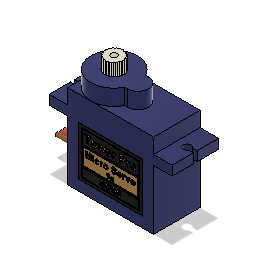
SG90 (Autodesk Fusion 360 design; units mm, degrees)
Autodesk Fusion 360 part; units mm, degrees
note: some values were not read from the file. Chosen so that the rebuilt part matches the saved one: which bodies a step acts on.
(part 1 of 2)
sketch "Sketch1" plane through (0, 0, 0) normal (0, 1, 0) x (1, 0, 0)
  line L0 (0, 0) -> (22.7, 0)
  line L1 (22.7, 0) -> (22.7, 12.3)
  line L2 (22.7, 12.3) -> (0, 12.3)
  line L3 (0, 12.3) -> (0, 0)
  dimension "d1" = 22.7
  dimension "d2" = 12.3
  constraint coincident L0.start L3.end
  constraint horizontal L0
  constraint perpendicular L0 L1
  constraint perpendicular L1 L2
  constraint perpendicular L0 L3
  measures "d1" distance of L0.start L0.end
  measures "d2" distance of L0.end L1.end
extrude "Extrude1" add sketch "Sketch1" along normal blind 22.3 makes body 1
sketch "Sketch2" plane through (0, 0, 0) normal (0, -1, 0) x (1, 0, 0)
  line L0 (0, 0) -> (0, -12.3)
  line L1 (0, -12.3) -> (22.7, -12.3)
  line L2 (22.7, -12.3) -> (22.7, 0)
  line L3 (22.7, 0) -> (0, 0)
  circle A0 centre (1.4, -1.7) radius 0.9
  circle A1 centre (1.4, -10.6) radius 0.9
  circle A2 centre (21.3, -1.7) radius 0.9
  circle A3 centre (21.3, -10.6) radius 0.9
  dimension "d9" = 1.8
  dimension "d10" = 1.8
  dimension "d11" = 1.8
  dimension "d12" = 1.8
  measures "d9" diameter of A0
  measures "d10" diameter of A1
  measures "d11" diameter of A2
  measures "d12" diameter of A3
extrude "Extrude2" cut sketch "Sketch2" against normal blind 1 contours A0 | A1 | A2 | A3 bodies 1
sketch "Sketch3" plane through (0, 1, 0) normal (0, -1, 0) x (1, 0, 0)
  circle A0 centre (1.4, -1.7) radius 0.9
  circle A1 centre (1.4, -1.7) radius 0.875
  dimension "d15" = 1.75
  constraint concentric A0 A1
  measures "d15" diameter of A1
extrude "Extrude3" add sketch "Sketch3" along normal blind 1 separate body contours A1 makes body 2
sketch "Sketch4" plane through (0, 0, 0) normal (0, -1, 0) x (1, 0, 0)
  circle A0 centre (1.4, -1.7) radius 0.875
  line L0 (1.9, -1.7) -> (1.9, -1.55)
  line L1 (0.9, -1.55) -> (0.9, -1.85)
  line L2 (1.9, -1.85) -> (1.9, -1.7)
  line L3 (1.4, -2.2) -> (1.55, -2.2)
  line L4 (1.55, -1.2) -> (1.25, -1.2)
  line L5 (1.25, -2.2) -> (1.4, -2.2)
  line L6 (0.9, -1.85) -> (1.25, -1.85)
  line L7 (1.55, -1.85) -> (1.9, -1.85)
  line L8 (1.25, -1.2) -> (1.25, -1.55)
  line L9 (1.25, -1.85) -> (1.25, -2.2)
  line L10 (1.9, -1.55) -> (1.55, -1.55)
  line L11 (1.25, -1.55) -> (0.9, -1.55)
  line L12 (1.55, -2.2) -> (1.55, -1.85)
  line L13 (1.55, -1.55) -> (1.55, -1.2)
  dimension "d18" = 0.15
  dimension "d19" = 0.3
  dimension "d20" = 0.15
  dimension "d21" = 0.3
  constraint perpendicular L0 L10
  constraint perpendicular L1 L10
  constraint perpendicular L1 L6
  constraint perpendicular L6 L12
  constraint perpendicular L4 L12
  constraint perpendicular L6 L8
  constraint coincident L6.end L8
  constraint collinear L6 L7
  constraint coincident L8.end L10
  constraint collinear L8 L9
  constraint coincident L10.end L12
  constraint collinear L10 L11
  constraint collinear L12 L13
  measures "d18" distance of L0.start L0.end
  measures "d19" distance of L1.start L1.end
  measures "d20" distance of L3.start L3.end
  measures "d21" distance of L4.start L4.end
extrude "Extrude4" cut sketch "Sketch4" against normal blind 0.5 contours L0 L1 L2 L3 L4 L5 L6 L7 L8 L9 L10 L11 L12 L13 bodies 2
fillet "Fillet1" radius 0.3 1 edges at (0.5842, 0, -2.0164) on bodies 2
pattern_linear "R-Pattern1" count 2 spacing 19.9 along (1, 0, 0) count 2 spacing 8.9 along (0, 0, -1) of bodies 2 makes body 3 at (20.721, 0.5333, -2.3561) makes body 4 at (2.2739, 0.5333, -10.6436) makes body 5 at (20.721, 0.5333, -11.2561)
sketch "Sketch5" plane through (0, 22.3, 0) normal (0, 1, 0) x (-1, 0, 0)
  line L0 (0, -12.3) -> (0, 0)
  line L1 (0, 0) -> (-22.7, 0)
  line L2 (-22.7, 0) -> (-22.7, -12.3)
  line L3 (-22.7, -12.3) -> (0, -12.3)
  line L4 (-12.45, -8.9) -> (-11.6509, -8.9)
  line L5 (-12.45, -3.4) -> (-11.6509, -3.4)
  arc A0 (-11.6509, -8.9) -> (-11.6509, -3.4) centre (-6.15, -6.15) ccw
  arc A1 (-12.45, -3.4) -> (-12.45, -8.9) centre (-12.45, -6.15) ccw
  line L6 (-12.3, -6.15) -> (-12.45, -6.15)
  dimension "d31" = 6.3
  dimension "d32" = 5.5
  constraint tangent L3 A0
  constraint coincident A1.centre L6.end
  constraint tangent L4 A1
  constraint tangent L5 A1
  measures "d31" distance of A0.centre A1.centre
  measures "d32" diameter of A1
extrude "Extrude5" add sketch "Sketch5" along normal blind 4.2 contours L4 L5 A0 A1 bodies 1
sketch "Sketch6" plane through (0, 26.5, 0) normal (0, 1, 0) x (-1, 0, 0)
  arc A0 (-12.45, -3.4) -> (-12.45, -8.9) centre (-12.45, -6.15) ccw
  line L0 (-12.45, -8.9) -> (-11.6509, -8.9)
  arc A1 (-11.6509, -8.9) -> (-11.6509, -3.4) centre (-6.15, -6.15) ccw
  line L1 (-11.6509, -3.4) -> (-12.45, -3.4)
  circle A2 centre (-6.15, -6.15) radius 2.5
  dimension "d35" = 5
  constraint concentric A1 A2
  measures "d35" diameter of A2
extrude "Extrude6" cut sketch "Sketch6" against normal blind 2 contours A2 bodies 1
sketch "Sketch7" plane through (0, 24.5, 0) normal (0, 1, 0) x (-1, 0, 0)
  circle A0 centre (-6.15, -6.15) radius 2.5
  line L0 (-6.15, -6.15) -> (-3.7, -6.15) construction
  line L1 (-5.8174, -8.3753) -> (-6.15, -8.6)
  line L2 (-6.15, -8.6) -> (-6.4826, -8.3753)
  line L3 (-5.1763, -8.1784) -> (-5.4278, -8.4912)
  line L4 (-5.4278, -8.4912) -> (-5.8119, -8.3744)
  line L5 (-4.6217, -7.8013) -> (-4.7699, -8.1743)
  line L6 (-4.7699, -8.1743) -> (-5.1712, -8.176)
  line L7 (-4.2028, -7.2774) -> (-4.2345, -7.6776)
  line L8 (-4.2345, -7.6776) -> (-4.6176, -7.7975)
  line L9 (-3.957, -6.6534) -> (-3.8694, -7.0451)
  line L10 (-3.8694, -7.0451) -> (-4.2, -7.2726)
  line L11 (-3.9061, -5.9847) -> (-3.7069, -6.3331)
  line L12 (-3.7069, -6.3331) -> (-3.9558, -6.6479)
  line L13 (-4.0545, -5.3306) -> (-3.7614, -5.6048)
  line L14 (-3.7614, -5.6048) -> (-3.9065, -5.9791)
  line L15 (-4.3891, -4.7493) -> (-4.0282, -4.925)
  line L16 (-4.0282, -4.925) -> (-4.0566, -5.3254)
  line L17 (-4.8802, -4.2925) -> (-4.4836, -4.354)
  line L18 (-4.4836, -4.354) -> (-4.3926, -4.745)
  line L19 (-5.4841, -4.0008) -> (-5.087, -3.9426)
  line L20 (-5.087, -3.9426) -> (-4.8848, -4.2894)
  line L21 (-6.1472, -3.9) -> (-5.7848, -3.7274)
  line L22 (-5.7848, -3.7274) -> (-5.4895, -3.9991)
  line L23 (-6.8105, -3.9991) -> (-6.5152, -3.7274)
  line L24 (-6.5152, -3.7274) -> (-6.1528, -3.9)
  line L25 (-7.4152, -4.2894) -> (-7.213, -3.9426)
  line L26 (-7.213, -3.9426) -> (-6.8159, -4.0008)
  line L27 (-7.9074, -4.745) -> (-7.8164, -4.354)
  line L28 (-7.8164, -4.354) -> (-7.4198, -4.2925)
  line L29 (-8.2434, -5.3254) -> (-8.2718, -4.925)
  line L30 (-8.2718, -4.925) -> (-7.9109, -4.7493)
  line L31 (-8.3935, -5.9791) -> (-8.5386, -5.6048)
  line L32 (-8.5386, -5.6048) -> (-8.2455, -5.3306)
  line L33 (-8.3442, -6.6479) -> (-8.5931, -6.3331)
  line L34 (-8.5931, -6.3331) -> (-8.3939, -5.9847)
  line L35 (-8.1, -7.2726) -> (-8.4306, -7.0451)
  line L36 (-8.4306, -7.0451) -> (-8.343, -6.6534)
  line L37 (-7.6824, -7.7975) -> (-8.0655, -7.6776)
  line L38 (-8.0655, -7.6776) -> (-8.0972, -7.2774)
  line L39 (-7.1288, -8.176) -> (-7.5301, -8.1743)
  line L40 (-7.5301, -8.1743) -> (-7.6783, -7.8013)
  line L41 (-6.4881, -8.3744) -> (-6.8722, -8.4912)
  line L42 (-6.8722, -8.4912) -> (-7.1237, -8.1784)
  arc A1 (-6.4881, -8.3744) -> (-6.4826, -8.3753) centre (-6.15, -6.15) ccw
  arc A2 (-7.1288, -8.176) -> (-7.1237, -8.1784) centre (-6.15, -6.15) ccw
  arc A3 (-7.6824, -7.7975) -> (-7.6783, -7.8013) centre (-6.15, -6.15) ccw
  arc A4 (-5.8174, -8.3753) -> (-5.8119, -8.3744) centre (-6.15, -6.15) ccw
  arc A5 (-5.1763, -8.1784) -> (-5.1712, -8.176) centre (-6.15, -6.15) ccw
  arc A6 (-4.6217, -7.8013) -> (-4.6176, -7.7975) centre (-6.15, -6.15) ccw
  arc A7 (-4.2028, -7.2774) -> (-4.2, -7.2726) centre (-6.15, -6.15) ccw
  arc A8 (-3.957, -6.6534) -> (-3.9558, -6.6479) centre (-6.15, -6.15) ccw
  arc A9 (-3.9061, -5.9847) -> (-3.9065, -5.9791) centre (-6.15, -6.15) ccw
  arc A10 (-4.0545, -5.3306) -> (-4.0566, -5.3254) centre (-6.15, -6.15) ccw
  arc A11 (-4.3891, -4.7493) -> (-4.3926, -4.745) centre (-6.15, -6.15) ccw
  arc A12 (-4.8802, -4.2925) -> (-4.8848, -4.2894) centre (-6.15, -6.15) ccw
  arc A13 (-5.4841, -4.0008) -> (-5.4895, -3.9991) centre (-6.15, -6.15) ccw
  arc A14 (-6.1472, -3.9) -> (-6.1528, -3.9) centre (-6.15, -6.15) ccw
  arc A15 (-6.8105, -3.9991) -> (-6.8159, -4.0008) centre (-6.15, -6.15) ccw
  arc A16 (-7.4152, -4.2894) -> (-7.4198, -4.2925) centre (-6.15, -6.15) ccw
  arc A17 (-7.9074, -4.745) -> (-7.9109, -4.7493) centre (-6.15, -6.15) ccw
  arc A18 (-8.2434, -5.3254) -> (-8.2455, -5.3306) centre (-6.15, -6.15) ccw
  arc A19 (-8.3935, -5.9791) -> (-8.3939, -5.9847) centre (-6.15, -6.15) ccw
  arc A20 (-8.3442, -6.6479) -> (-8.343, -6.6534) centre (-6.15, -6.15) ccw
  arc A21 (-8.1, -7.2726) -> (-8.0972, -7.2774) centre (-6.15, -6.15) ccw
  dimension "d39" = 4.5
  dimension "d43" = 360
  constraint concentric A0 A4
  constraint horizontal L0
  constraint concentric A1 A4
  constraint concentric A2 A4
  constraint concentric A3 A4
  constraint concentric A4 A5
  constraint concentric A5 A6
  constraint concentric A6 A7
  constraint concentric A7 A8
  constraint concentric A8 A9
  constraint concentric A9 A10
  constraint concentric A10 A11
  constraint concentric A11 A12
  constraint concentric A12 A13
  constraint concentric A13 A14
  constraint concentric A14 A15
  constraint concentric A15 A16
  constraint concentric A16 A17
  constraint concentric A17 A18
  constraint concentric A18 A19
  constraint concentric A19 A20
  constraint concentric A20 A21
  measures "d39" diameter of A4
extrude "Extrude7" add sketch "Sketch7" along normal blind 5.2 separate body contours L1 L2 L3 L4 L5 L6 L7 L8 L9 L10 L11 L12 L13 L14 L15 L16 L17 L18 L19 L20 L21 L22 L23 L24 L25 L26 L27 L28 L29 L30 L31 L32 L33 L34 L35 L36 L37 L38 L39 L40 L41 L42 A1 A2 A3 A4 A5 A6 A7 A8 A9 A10 A11 A12 A13 A14 A15 A16 A17 A18 A19 A20 A21 makes body 6
sketch "Sketch8" plane through (0, 29.7, 0) normal (0, 1, 0) x (-1, 0, 0)
  line L0 (-8.4306, -7.0451) -> (-8.1, -7.2726)
  arc A0 (-8.1, -7.2726) -> (-8.0972, -7.2774) centre (-6.15, -6.15) ccw
  line L1 (-8.0972, -7.2774) -> (-8.0655, -7.6776)
  line L2 (-8.0655, -7.6776) -> (-7.6824, -7.7975)
  arc A1 (-7.6824, -7.7975) -> (-7.6783, -7.8013) centre (-6.15, -6.15) ccw
  line L3 (-7.6783, -7.8013) -> (-7.5301, -8.1743)
  line L4 (-7.5301, -8.1743) -> (-7.1288, -8.176)
  arc A2 (-7.1288, -8.176) -> (-7.1237, -8.1784) centre (-6.15, -6.15) ccw
  line L5 (-7.1237, -8.1784) -> (-6.8722, -8.4912)
  line L6 (-6.8722, -8.4912) -> (-6.4881, -8.3744)
  arc A3 (-6.4881, -8.3744) -> (-6.4826, -8.3753) centre (-6.15, -6.15) ccw
  line L7 (-6.4826, -8.3753) -> (-6.15, -8.6)
  line L8 (-6.15, -8.6) -> (-5.8174, -8.3753)
  arc A4 (-5.8174, -8.3753) -> (-5.8119, -8.3744) centre (-6.15, -6.15) ccw
  line L9 (-5.8119, -8.3744) -> (-5.4278, -8.4912)
  line L10 (-5.4278, -8.4912) -> (-5.1763, -8.1784)
  arc A5 (-5.1763, -8.1784) -> (-5.1712, -8.176) centre (-6.15, -6.15) ccw
  line L11 (-5.1712, -8.176) -> (-4.7699, -8.1743)
  line L12 (-4.7699, -8.1743) -> (-4.6217, -7.8013)
  arc A6 (-4.6217, -7.8013) -> (-4.6176, -7.7975) centre (-6.15, -6.15) ccw
  line L13 (-4.6176, -7.7975) -> (-4.2345, -7.6776)
  line L14 (-4.2345, -7.6776) -> (-4.2028, -7.2774)
  arc A7 (-4.2028, -7.2774) -> (-4.2, -7.2726) centre (-6.15, -6.15) ccw
  line L15 (-4.2, -7.2726) -> (-3.8694, -7.0451)
  line L16 (-3.8694, -7.0451) -> (-3.957, -6.6534)
  arc A8 (-3.957, -6.6534) -> (-3.9558, -6.6479) centre (-6.15, -6.15) ccw
  line L17 (-3.9558, -6.6479) -> (-3.7069, -6.3331)
  line L18 (-3.7069, -6.3331) -> (-3.9061, -5.9847)
  arc A9 (-3.9061, -5.9847) -> (-3.9065, -5.9791) centre (-6.15, -6.15) ccw
  line L19 (-3.9065, -5.9791) -> (-3.7614, -5.6048)
  line L20 (-3.7614, -5.6048) -> (-4.0545, -5.3306)
  arc A10 (-4.0545, -5.3306) -> (-4.0566, -5.3254) centre (-6.15, -6.15) ccw
  line L21 (-4.0566, -5.3254) -> (-4.0282, -4.925)
  line L22 (-4.0282, -4.925) -> (-4.3891, -4.7493)
  arc A11 (-4.3891, -4.7493) -> (-4.3926, -4.745) centre (-6.15, -6.15) ccw
  line L23 (-4.3926, -4.745) -> (-4.4836, -4.354)
  line L24 (-4.4836, -4.354) -> (-4.8802, -4.2925)
  arc A12 (-4.8802, -4.2925) -> (-4.8848, -4.2894) centre (-6.15, -6.15) ccw
  line L25 (-4.8848, -4.2894) -> (-5.087, -3.9426)
  line L26 (-5.087, -3.9426) -> (-5.4841, -4.0008)
  arc A13 (-5.4841, -4.0008) -> (-5.4895, -3.9991) centre (-6.15, -6.15) ccw
  line L27 (-5.4895, -3.9991) -> (-5.7848, -3.7274)
  line L28 (-5.7848, -3.7274) -> (-6.1472, -3.9)
  arc A14 (-6.1472, -3.9) -> (-6.1528, -3.9) centre (-6.15, -6.15) ccw
  line L29 (-6.1528, -3.9) -> (-6.5152, -3.7274)
  line L30 (-6.5152, -3.7274) -> (-6.8105, -3.9991)
  arc A15 (-6.8105, -3.9991) -> (-6.8159, -4.0008) centre (-6.15, -6.15) ccw
  line L31 (-6.8159, -4.0008) -> (-7.213, -3.9426)
  line L32 (-7.213, -3.9426) -> (-7.4152, -4.2894)
  arc A16 (-7.4152, -4.2894) -> (-7.4198, -4.2925) centre (-6.15, -6.15) ccw
  line L33 (-7.4198, -4.2925) -> (-7.8164, -4.354)
  line L34 (-7.8164, -4.354) -> (-7.9074, -4.745)
  arc A17 (-7.9074, -4.745) -> (-7.9109, -4.7493) centre (-6.15, -6.15) ccw
  line L35 (-7.9109, -4.7493) -> (-8.2718, -4.925)
  line L36 (-8.2718, -4.925) -> (-8.2434, -5.3254)
  arc A18 (-8.2434, -5.3254) -> (-8.2455, -5.3306) centre (-6.15, -6.15) ccw
  line L37 (-8.2455, -5.3306) -> (-8.5386, -5.6048)
  line L38 (-8.5386, -5.6048) -> (-8.3935, -5.9791)
  arc A19 (-8.3935, -5.9791) -> (-8.3939, -5.9847) centre (-6.15, -6.15) ccw
  line L39 (-8.3939, -5.9847) -> (-8.5931, -6.3331)
  line L40 (-8.5931, -6.3331) -> (-8.3442, -6.6479)
  arc A20 (-8.3442, -6.6479) -> (-8.343, -6.6534) centre (-6.15, -6.15) ccw
  line L41 (-8.343, -6.6534) -> (-8.4306, -7.0451)
  circle A21 centre (-6.15, -6.15) radius 0.8
  dimension "d46" = 1.6
  constraint concentric A0 A21
  measures "d46" diameter of A21
extrude "Extrude8" cut sketch "Sketch8" against normal blind 4 contours A21 bodies 6
sketch "Sketch9" plane through (22.7, 0, 0) normal (1, 0, 0) x (0, 0, -1)
  line L0 (0, 0) -> (12.3, 0)
  line L1 (12.3, 0) -> (12.3, 22.3)
  line L2 (12.3, 22.3) -> (0, 22.3)
  line L3 (0, 22.3) -> (0, 0)
  line L4 (12.3, 22.3) -> (12.3, 15.8)
  line L5 (12.3, 15.8) -> (0, 15.8)
  line L6 (0, 15.8) -> (0, 18.3)
  line L7 (0, 18.3) -> (12.3, 18.3256)
  line L8 (12.3, 18.3256) -> (12.3, 15.8)
  dimension "d49" = 6.5
  dimension "d50" = 2.5
  constraint coincident L1.end L2.start
  constraint perpendicular L2 L4
  constraint coincident L3 L5.end
  constraint perpendicular L3 L5
  constraint perpendicular L5 L6
  constraint coincident L1 L7.end
  measures "d49" distance of L1.end L4.end
  measures "d50" distance of L5.end L6.end
extrude "Extrude9" add sketch "Sketch9" along normal blind 4.9 contours L1 L3 L4 L5 L6 L7 L8 bodies 1
sketch "Sketch10" plane through (0, 18.2999, 0.038) normal (0, 0.999998, 0.002078) x (1, 0, 0)
  line L0 (22.7, 12.3381) -> (22.7, 0.038)
  line L1 (22.7, 0.038) -> (27.6, 0.038)
  line L2 (27.6, 0.038) -> (27.6, 12.3381)
  line L3 (27.6, 12.3381) -> (22.7, 12.3381)
  line L4 (27.6, 6.188) -> (27.6, 6.688)
  line L5 (27.6, 6.688) -> (26.316, 6.688)
  line L6 (27.6, 6.188) -> (27.6, 5.688)
  line L7 (27.6, 5.688) -> (26.316, 5.688)
  arc A0 (26.316, 6.688) -> (26.316, 5.688) centre (25.45, 6.188) ccw
  dimension "d53" = 2.15
  dimension "d54" = 2
  dimension "d55" = 0.5
  dimension "d56" = 0.5
  constraint midpoint L2 L4.start
  constraint perpendicular L4 L5
  constraint perpendicular L2 L7
  measures "d53" distance of L4.start A0.centre
  measures "d54" diameter of A0
  measures "d55" distance of L4.start L4.end
  measures "d56" distance of L4.start L6.end
extrude "Extrude10" cut sketch "Sketch10" against normal blind 7 contours L2 L4 L5 L6 L7 A0 bodies 1
sketch "Sketch11" plane through (0, 15.8, 0) normal (0, -1, 0) x (1, 0, 0)
  line L0 (26.316, -5.6552) -> (27.6, -5.6552)
  line L1 (27.6, -5.6552) -> (27.6, 0)
  line L2 (27.6, 0) -> (22.7, 0)
  line L3 (22.7, 0) -> (22.7, -12.3)
  line L4 (22.7, -12.3) -> (27.6, -12.3)
  line L5 (27.6, -12.3) -> (27.6, -6.6552)
  line L6 (27.6, -6.6552) -> (26.316, -6.6552)
  ellipse E0 centre (25.45, -6.1552) end of major axis (25.45, -7.1552) minor radius 1 (26.316, -5.6552) -> (26.316, -6.6552) ccw
  line L7 (23.7, -1) -> (22.7, -1)
  line L8 (23.7, -11.3) -> (22.7, -11.3)
  spline S0 degree 3 poles (23.7, -7.1235) (23.7918, -7.2893) (23.908, -7.443) (24.0431, -7.5767) (24.5836, -8.1117) (25.4438, -8.2949) (26.1554, -8.0267) (26.3127, -7.9674) (26.4625, -7.8882) (26.6, -7.7915) knots 5.21775 5.21775 5.21775 5.21775 5.502936 5.502936 5.502936 6.643656 6.643656 6.643656 6.895789 6.895789 6.895789 6.895789
  line L9 (26.6, -11.3) -> (26.6, -7.7915)
  spline S1 degree 3 poles (26.6, -4.5189) (26.2218, -4.2531) (25.748, -4.1241) (25.2866, -4.1619) (24.633, -4.2155) (24.0163, -4.6152) (23.7, -5.187) knots 2.528989 2.528989 2.528989 2.528989 3.223367 3.223367 3.223367 4.207028 4.207028 4.207028 4.207028
  line L10 (26.6, -1) -> (23.7, -1)
  line L11 (26.6, -4.5189) -> (26.6, -1)
  arc A0 (26.6, -4.5189) -> (26.6, -7.7915) centre (25.45, -6.1552) ccw
  line L12 (23.7, -11.3) -> (26.6, -11.3)
  line L13 (22.7, -11.3) -> (22.7, -1)
  constraint coincident L3 L7.end
  constraint perpendicular L3 L7
  constraint coincident L3 L8.end
  constraint perpendicular L3 L8
  constraint perpendicular L9 L12
extrude "Extrude11" cut sketch "Sketch11" against normal blind 1 contours L3 L7 L8 S0 L9 S1 L10 L11 A0 L12 L13 bodies 1
ref_plane "WorkPlane1" through (11.35, 0, 0) normal (1, 0, 0) x (0, 1, 0)
mirror "Mirror1" about plane through (11.35, 0, 0) normal (1, 0, 0) of "Extrude9"
mirror "Mirror2" about plane through (11.35, 0, 0) normal (1, 0, 0) of "Extrude10"
mirror "Mirror3" about plane through (11.35, 0, 0) normal (1, 0, 0) of "Extrude11"
sketch "Sketch12" plane through (0, 0, 0) normal (0, 0, 1) x (1, 0, 0)
  line L0 (0, 0) -> (22.7, 0)
  line L1 (22.7, 0) -> (22.7, 15.8)
  line L2 (22.7, 15.8) -> (27.6, 15.8)
  line L3 (27.6, 15.8) -> (27.6, 18.3)
  line L4 (27.6, 18.3) -> (22.7, 18.3)
  line L5 (22.7, 18.3) -> (22.7, 22.3)
  line L6 (22.7, 22.3) -> (6.15, 22.3)
  line L7 (6.15, 22.3) -> (0, 22.3)
  line L8 (0, 22.3) -> (0, 18.3)
  line L9 (0, 18.3) -> (-4.9, 18.3)
  line L10 (-4.9, 18.3) -> (-4.9, 15.8)
  line L11 (-4.9, 15.8) -> (0, 15.8)
  line L12 (0, 15.8) -> (0, 0)
  line L13 (11.35, 0) -> (19.85, 0)
  line L14 (19.85, 15.8) -> (2.85, 15.8)
  line L15 (19.85, 15.8) -> (19.85, 2.8)
  line L16 (19.85, 2.8) -> (2.85, 2.8)
  line L17 (2.85, 2.8) -> (2.85, 15.8)
  dimension "d69" = 8.5
  dimension "d70" = 13
  dimension "d71" = 17
  constraint midpoint L0 L13.start
  constraint parallel L0 L13
  constraint perpendicular L14 L15
  constraint perpendicular L15 L16
  constraint perpendicular L14 L17
  measures "d69" distance of L13.start L13.end
  measures "d70" distance of L14.start L15.end
  measures "d71" distance of L15.end L16.end
extrude "Extrude12" add sketch "Sketch12" along normal blind 0.05 separate body contours L14 L15 L16 L17 makes body 7
sketch "Sketch13" plane through (0, 0, 0.05) normal (0, 0, 1) x (1, 0, 0)
  line L0 (19.85, 15.8) -> (2.85, 15.8)
  line L1 (2.85, 15.8) -> (2.85, 2.8)
  line L2 (2.85, 2.8) -> (19.85, 2.8)
  line L3 (19.85, 2.8) -> (19.85, 15.8)
  line L4 (19.05, 9.3) -> (19.05, 15.05)
  line L5 (19.05, 15.05) -> (3.65, 15.05)
  line L6 (3.65, 15.05) -> (3.65, 3.55)
  line L7 (3.65, 3.55) -> (19.05, 3.55)
  line L8 (19.05, 3.55) -> (19.05, 9.3)
  line L9 (3.65, 15.05) -> (3.85, 15.05)
  line L10 (3.85, 3.75) -> (18.85, 3.75)
  line L11 (18.85, 14.85) -> (3.85, 14.85)
  line L12 (3.85, 14.85) -> (3.85, 11.35)
  line L13 (3.85, 11.35) -> (18.85, 11.35)
  line L14 (18.85, 11.15) -> (3.85, 11.15)
  line L15 (3.85, 14.85) -> (3.85, 11.35)
  line L16 (18.85, 11.35) -> (18.85, 14.85)
  line L17 (18.85, 3.75) -> (18.85, 6.05)
  line L18 (18.85, 6.05) -> (3.85, 6.05)
  line L19 (3.85, 6.25) -> (18.85, 6.25)
  line L20 (18.85, 3.75) -> (18.85, 6.05)
  line L21 (18.85, 6.25) -> (18.85, 11.15)
  line L22 (3.85, 11.15) -> (3.85, 6.25)
  line L23 (3.85, 6.05) -> (3.85, 3.75)
  line L24 (3.85, 11.15) -> (4.15, 11.15)
  line L25 (4.15, 10.85) -> (4.15, 6.55)
  line L26 (4.15, 10.85) -> (18.55, 10.85)
  line L27 (18.55, 10.85) -> (18.55, 6.55)
  line L28 (18.55, 6.55) -> (4.15, 6.55)
  dimension "d75" = 5.75
  dimension "d76" = 15.4
  dimension "d77" = 11.5
  dimension "d78" = 15.4
  dimension "d79" = 0.2
  dimension "d83" = 3.5
  dimension "d84" = 0.2
  dimension "d85" = 2.3
  dimension "d86" = 0.2
  dimension "d87" = 0.3
  dimension "d88" = 0.3
  constraint perpendicular L4 L5
  constraint perpendicular L5 L6
  constraint perpendicular L6 L7
  constraint horizontal L9
  constraint perpendicular L7 L15
  constraint perpendicular L8 L10
  constraint perpendicular L5 L20
  constraint perpendicular L11 L15
  constraint perpendicular L11 L12
  constraint coincident L13.end L20
  constraint perpendicular L13 L20
  constraint coincident L14.end L15
  constraint perpendicular L14 L15
  constraint collinear L15 L22
  constraint collinear L16 L20
  constraint perpendicular L10 L17
  constraint coincident L18.end L22
  constraint perpendicular L18 L22
  constraint coincident L19.end L20
  constraint perpendicular L19 L20
  constraint collinear L20 L21
  constraint collinear L22 L23
  constraint perpendicular L22 L24
  constraint perpendicular L19 L25
  constraint perpendicular L21 L26
  constraint perpendicular L19 L27
  constraint perpendicular L25 L28
  measures "d75" distance of L4.start L4.end
  measures "d76" distance of L4.end L5.end
  measures "d77" distance of L5.end L6.end
  measures "d78" distance of L6.end L7.end
  measures "d79" distance of L5.end L9.end
  measures "d83" distance of L11.end L12.end
  measures "d84" distance of L13.end L14.start
  measures "d85" distance of L10.end L17.end
  measures "d86" distance of L18.end L19.start
  measures "d87" distance of L14.end L24.end
  measures "d88" distance of L24.end L25.start
extrude "Extrude13" add sketch "Sketch13" along normal blind 0.05 contours L4 L5 L6 L7 L8 L9 | L25 L26 L27 L28 bodies 7
sketch "Sketch14" plane through (0, 0, 0.05) normal (0, 0, 1) x (1, 0, 0)
  line L0 (18.85, 14.85) -> (3.85, 14.85)
  line L1 (3.85, 14.85) -> (3.85, 11.35)
  line L2 (3.85, 11.35) -> (18.85, 11.35)
  line L3 (18.85, 11.35) -> (18.85, 14.85)
  line L4 (5.1924, 12.1) -> (5.1924, 13.7617)
  line L5 (5.1924, 13.7617) -> (4.599, 13.7617)
  line L6 (4.599, 13.7617) -> (4.599, 14.1)
  line L7 (4.599, 14.1) -> (6.1883, 14.1)
  line L8 (6.1883, 14.1) -> (6.1883, 13.7617)
  line L9 (6.1883, 13.7617) -> (5.5962, 13.7617)
  line L10 (5.5962, 13.7617) -> (5.5962, 12.1)
  line L11 (5.5962, 12.1) -> (5.1924, 12.1)
  spline S0 degree 2 poles (6.3575, 12.8449) (6.3575, 13.0359) (6.4516, 13.2146) knots 0 0 0 1 1 1
  spline S1 degree 2 poles (6.4516, 13.2146) (6.5458, 13.3933) (6.7177, 13.4874) knots 0 0 0 1 1 1
  spline S2 degree 2 poles (6.7177, 13.4874) (6.8909, 13.5816) (7.1038, 13.5816) knots 0 0 0 1 1 1
  spline S3 degree 2 poles (7.1038, 13.5816) (7.4325, 13.5816) (7.6426, 13.3674) knots 0 0 0 1 1 1
  spline S4 degree 2 poles (7.6426, 13.3674) (7.8527, 13.1546) (7.8527, 12.8285) knots 0 0 0 1 1 1
  spline S5 degree 2 poles (7.8527, 12.8285) (7.8527, 12.4997) (7.6399, 12.2828) knots 0 0 0 1 1 1
  spline S6 degree 2 poles (7.6399, 12.2828) (7.4284, 12.0673) (7.1065, 12.0673) knots 0 0 0 1 1 1
  spline S7 degree 2 poles (7.1065, 12.0673) (6.9073, 12.0673) (6.7259, 12.1573) knots 0 0 0 1 1 1
  spline S8 degree 2 poles (6.7259, 12.1573) (6.5458, 12.2473) (6.4516, 12.4206) knots 0 0 0 1 1 1
  spline S9 degree 2 poles (6.4516, 12.4206) (6.3575, 12.5952) (6.3575, 12.8449) knots 0 0 0 1 1 1
  spline S10 degree 2 poles (6.7504, 12.8244) (6.7504, 12.6089) (6.8527, 12.4943) knots 0 0 0 1 1 1
  spline S11 degree 2 poles (6.8527, 12.4943) (6.955, 12.3797) (7.1051, 12.3797) knots 0 0 0 1 1 1
  spline S12 degree 2 poles (7.1051, 12.3797) (7.2552, 12.3797) (7.3561, 12.4943) knots 0 0 0 1 1 1
  spline S13 degree 2 poles (7.3561, 12.4943) (7.4585, 12.6089) (7.4585, 12.8271) knots 0 0 0 1 1 1
  spline S14 degree 2 poles (7.4585, 12.8271) (7.4585, 13.04) (7.3561, 13.1546) knots 0 0 0 1 1 1
  spline S15 degree 2 poles (7.3561, 13.1546) (7.2552, 13.2692) (7.1051, 13.2692) knots 0 0 0 1 1 1
  spline S16 degree 2 poles (7.1051, 13.2692) (6.955, 13.2692) (6.8527, 13.1546) knots 0 0 0 1 1 1
  spline S17 degree 2 poles (6.8527, 13.1546) (6.7504, 13.04) (6.7504, 12.8244) knots 0 0 0 1 1 1
  line L12 (8.423, 12.1) -> (7.9646, 13.5488)
  line L13 (7.9646, 13.5488) -> (8.337, 13.5488)
  line L14 (8.337, 13.5488) -> (8.6085, 12.5993)
  line L15 (8.6085, 12.5993) -> (8.8582, 13.5488)
  line L16 (8.8582, 13.5488) -> (9.2279, 13.5488)
  line L17 (9.2279, 13.5488) -> (9.4694, 12.5993)
  line L18 (9.4694, 12.5993) -> (9.7463, 13.5488)
  line L19 (9.7463, 13.5488) -> (10.1242, 13.5488)
  line L20 (10.1242, 13.5488) -> (9.659, 12.1)
  line L21 (9.659, 12.1) -> (9.2907, 12.1)
  line L22 (9.2907, 12.1) -> (9.041, 13.0318)
  line L23 (9.041, 13.0318) -> (8.7954, 12.1)
  line L24 (8.7954, 12.1) -> (8.423, 12.1)
  line L25 (11.1651, 12.5611) -> (11.5471, 12.497)
  spline S18 degree 2 poles (11.5471, 12.497) (11.4735, 12.2869) (11.3138, 12.1764) knots 0 0 0 1 1 1
  spline S19 degree 2 poles (11.3138, 12.1764) (11.1556, 12.0673) (10.9168, 12.0673) knots 0 0 0 1 1 1
  spline S20 degree 2 poles (10.9168, 12.0673) (10.5389, 12.0673) (10.3575, 12.3142) knots 0 0 0 1 1 1
  spline S21 degree 2 poles (10.3575, 12.3142) (10.2143, 12.512) (10.2143, 12.8135) knots 0 0 0 1 1 1
  spline S22 degree 2 poles (10.2143, 12.8135) (10.2143, 13.1737) (10.4025, 13.3769) knots 0 0 0 1 1 1
  spline S23 degree 2 poles (10.4025, 13.3769) (10.5908, 13.5816) (10.8786, 13.5816) knots 0 0 0 1 1 1
  spline S24 degree 2 poles (10.8786, 13.5816) (11.202, 13.5816) (11.3889, 13.3674) knots 0 0 0 1 1 1
  spline S25 degree 2 poles (11.3889, 13.3674) (11.5758, 13.1546) (11.5676, 12.7139) knots 0 0 0 1 1 1
  line L26 (11.5676, 12.7139) -> (10.6072, 12.7139)
  spline S26 degree 2 poles (10.6072, 12.7139) (10.6113, 12.5434) (10.6999, 12.4479) knots 0 0 0 1 1 1
  spline S27 degree 2 poles (10.6999, 12.4479) (10.7886, 12.3538) (10.9209, 12.3538) knots 0 0 0 1 1 1
  spline S28 degree 2 poles (10.9209, 12.3538) (11.011, 12.3538) (11.0724, 12.4029) knots 0 0 0 1 1 1
  spline S29 degree 2 poles (11.0724, 12.4029) (11.1338, 12.452) (11.1651, 12.5611) knots 0 0 0 1 1 1
  spline S30 degree 2 poles (11.187, 12.9486) (11.1829, 13.115) (11.101, 13.201) knots 0 0 0 1 1 1
  spline S31 degree 2 poles (11.101, 13.201) (11.0192, 13.2883) (10.9018, 13.2883) knots 0 0 0 1 1 1
  spline S32 degree 2 poles (10.9018, 13.2883) (10.7763, 13.2883) (10.6945, 13.1969) knots 0 0 0 1 1 1
  spline S33 degree 2 poles (10.6945, 13.1969) (10.6126, 13.1055) (10.614, 12.9486) knots 0 0 0 1 1 1
  line L27 (10.614, 12.9486) -> (11.187, 12.9486)
  line L28 (12.247, 12.1) -> (11.8636, 12.1)
  line L29 (11.8636, 12.1) -> (11.8636, 13.5488)
  line L30 (11.8636, 13.5488) -> (12.2197, 13.5488)
  line L31 (12.2197, 13.5488) -> (12.2197, 13.3428)
  spline S34 degree 2 poles (12.2197, 13.3428) (12.3111, 13.4888) (12.3834, 13.5352) knots 0 0 0 1 1 1
  spline S35 degree 2 poles (12.3834, 13.5352) (12.4571, 13.5816) (12.5499, 13.5816) knots 0 0 0 1 1 1
  spline S36 degree 2 poles (12.5499, 13.5816) (12.6808, 13.5816) (12.8023, 13.5093) knots 0 0 0 1 1 1
  line L32 (12.8023, 13.5093) -> (12.6836, 13.175)
  spline S37 degree 2 poles (12.6836, 13.175) (12.5867, 13.2378) (12.5035, 13.2378) knots 0 0 0 1 1 1
  spline S38 degree 2 poles (12.5035, 13.2378) (12.423, 13.2378) (12.3671, 13.1928) knots 0 0 0 1 1 1
  spline S39 degree 2 poles (12.3671, 13.1928) (12.3111, 13.1491) (12.2784, 13.0332) knots 0 0 0 1 1 1
  spline S40 degree 2 poles (12.2784, 13.0332) (12.247, 12.9172) (12.247, 12.5475) knots 0 0 0 1 1 1
  line L33 (12.247, 12.5475) -> (12.247, 12.1)
  line L34 (13.7463, 12.1) -> (13.7463, 14.1)
  line L35 (13.7463, 14.1) -> (14.3943, 14.1)
  spline S41 degree 2 poles (14.3943, 14.1) (14.7627, 14.1) (14.8746, 14.07) knots 0 0 0 1 1 1
  spline S42 degree 2 poles (14.8746, 14.07) (15.0465, 14.025) (15.1624, 13.8735) knots 0 0 0 1 1 1
  spline S43 degree 2 poles (15.1624, 13.8735) (15.2784, 13.7235) (15.2784, 13.4847) knots 0 0 0 1 1 1
  spline S44 degree 2 poles (15.2784, 13.4847) (15.2784, 13.3005) (15.2115, 13.175) knots 0 0 0 1 1 1
  spline S45 degree 2 poles (15.2115, 13.175) (15.1447, 13.0495) (15.041, 12.9772) knots 0 0 0 1 1 1
  spline S46 degree 2 poles (15.041, 12.9772) (14.9387, 12.9063) (14.8323, 12.8831) knots 0 0 0 1 1 1
  spline S47 degree 2 poles (14.8323, 12.8831) (14.6877, 12.8544) (14.4134, 12.8544) knots 0 0 0 1 1 1
  line L36 (14.4134, 12.8544) -> (14.1501, 12.8544)
  line L37 (14.1501, 12.8544) -> (14.1501, 12.1)
  line L38 (14.1501, 12.1) -> (13.7463, 12.1)
  line L39 (14.1501, 13.7617) -> (14.1501, 13.1941)
  line L40 (14.1501, 13.1941) -> (14.3711, 13.1941)
  spline S48 degree 2 poles (14.3711, 13.1941) (14.6099, 13.1941) (14.6904, 13.2255) knots 0 0 0 1 1 1
  spline S49 degree 2 poles (14.6904, 13.2255) (14.7709, 13.2569) (14.8159, 13.3237) knots 0 0 0 1 1 1
  spline S50 degree 2 poles (14.8159, 13.3237) (14.8623, 13.3906) (14.8623, 13.4793) knots 0 0 0 1 1 1
  spline S51 degree 2 poles (14.8623, 13.4793) (14.8623, 13.5884) (14.7982, 13.6593) knots 0 0 0 1 1 1
  spline S52 degree 2 poles (14.7982, 13.6593) (14.734, 13.7303) (14.6358, 13.748) knots 0 0 0 1 1 1
  spline S53 degree 2 poles (14.6358, 13.748) (14.5635, 13.7617) (14.3452, 13.7617) knots 0 0 0 1 1 1
  line L41 (14.3452, 13.7617) -> (14.1501, 13.7617)
  line L42 (15.9741, 12.1) -> (15.5908, 12.1)
  line L43 (15.5908, 12.1) -> (15.5908, 13.5488)
  line L44 (15.5908, 13.5488) -> (15.9469, 13.5488)
  line L45 (15.9469, 13.5488) -> (15.9469, 13.3428)
  spline S54 degree 2 poles (15.9469, 13.3428) (16.0383, 13.4888) (16.1106, 13.5352) knots 0 0 0 1 1 1
  spline S55 degree 2 poles (16.1106, 13.5352) (16.1842, 13.5816) (16.277, 13.5816) knots 0 0 0 1 1 1
  spline S56 degree 2 poles (16.277, 13.5816) (16.408, 13.5816) (16.5294, 13.5093) knots 0 0 0 1 1 1
  line L46 (16.5294, 13.5093) -> (16.4107, 13.175)
  spline S57 degree 2 poles (16.4107, 13.175) (16.3138, 13.2378) (16.2306, 13.2378) knots 0 0 0 1 1 1
  spline S58 degree 2 poles (16.2306, 13.2378) (16.1501, 13.2378) (16.0942, 13.1928) knots 0 0 0 1 1 1
  spline S59 degree 2 poles (16.0942, 13.1928) (16.0383, 13.1491) (16.0055, 13.0332) knots 0 0 0 1 1 1
  spline S60 degree 2 poles (16.0055, 13.0332) (15.9741, 12.9172) (15.9741, 12.5475) knots 0 0 0 1 1 1
  line L47 (15.9741, 12.5475) -> (15.9741, 12.1)
  spline S61 degree 2 poles (16.6058, 12.8449) (16.6058, 13.0359) (16.6999, 13.2146) knots 0 0 0 1 1 1
  spline S62 degree 2 poles (16.6999, 13.2146) (16.7941, 13.3933) (16.966, 13.4874) knots 0 0 0 1 1 1
  spline S63 degree 2 poles (16.966, 13.4874) (17.1392, 13.5816) (17.352, 13.5816) knots 0 0 0 1 1 1
  spline S64 degree 2 poles (17.352, 13.5816) (17.6808, 13.5816) (17.8909, 13.3674) knots 0 0 0 1 1 1
  spline S65 degree 2 poles (17.8909, 13.3674) (18.101, 13.1546) (18.101, 12.8285) knots 0 0 0 1 1 1
  spline S66 degree 2 poles (18.101, 12.8285) (18.101, 12.4997) (17.8882, 12.2828) knots 0 0 0 1 1 1
  spline S67 degree 2 poles (17.8882, 12.2828) (17.6767, 12.0673) (17.3548, 12.0673) knots 0 0 0 1 1 1
  spline S68 degree 2 poles (17.3548, 12.0673) (17.1556, 12.0673) (16.9741, 12.1573) knots 0 0 0 1 1 1
  spline S69 degree 2 poles (16.9741, 12.1573) (16.7941, 12.2473) (16.6999, 12.4206) knots 0 0 0 1 1 1
  spline S70 degree 2 poles (16.6999, 12.4206) (16.6058, 12.5952) (16.6058, 12.8449) knots 0 0 0 1 1 1
  spline S71 degree 2 poles (16.9987, 12.8244) (16.9987, 12.6089) (17.101, 12.4943) knots 0 0 0 1 1 1
  spline S72 degree 2 poles (17.101, 12.4943) (17.2033, 12.3797) (17.3534, 12.3797) knots 0 0 0 1 1 1
  spline S73 degree 2 poles (17.3534, 12.3797) (17.5035, 12.3797) (17.6044, 12.4943) knots 0 0 0 1 1 1
  spline S74 degree 2 poles (17.6044, 12.4943) (17.7068, 12.6089) (17.7068, 12.8271) knots 0 0 0 1 1 1
  spline S75 degree 2 poles (17.7068, 12.8271) (17.7068, 13.04) (17.6044, 13.1546) knots 0 0 0 1 1 1
  spline S76 degree 2 poles (17.6044, 13.1546) (17.5035, 13.2692) (17.3534, 13.2692) knots 0 0 0 1 1 1
  spline S77 degree 2 poles (17.3534, 13.2692) (17.2033, 13.2692) (17.101, 13.1546) knots 0 0 0 1 1 1
  spline S78 degree 2 poles (17.101, 13.1546) (16.9987, 13.04) (16.9987, 12.8244) knots 0 0 0 1 1 1
  line L48 (8.5877, 4.6206) -> (8.902, 4.6512)
  spline S79 degree 2 poles (8.902, 4.6512) (8.9304, 4.4929) (9.0166, 4.4187) knots 0 0 0 1 1 1
  spline S80 degree 2 poles (9.0166, 4.4187) (9.1039, 4.3445) (9.2512, 4.3445) knots 0 0 0 1 1 1
  spline S81 degree 2 poles (9.2512, 4.3445) (9.4073, 4.3445) (9.4859, 4.41) knots 0 0 0 1 1 1
  spline S82 degree 2 poles (9.4859, 4.41) (9.5656, 4.4765) (9.5656, 4.5649) knots 0 0 0 1 1 1
  spline S83 degree 2 poles (9.5656, 4.5649) (9.5656, 4.6217) (9.5317, 4.661) knots 0 0 0 1 1 1
  spline S84 degree 2 poles (9.5317, 4.661) (9.499, 4.7014) (9.416, 4.7308) knots 0 0 0 1 1 1
  spline S85 degree 2 poles (9.416, 4.7308) (9.3593, 4.7505) (9.1574, 4.8007) knots 0 0 0 1 1 1
  spline S86 degree 2 poles (9.1574, 4.8007) (8.8976, 4.8651) (8.7928, 4.9589) knots 0 0 0 1 1 1
  spline S87 degree 2 poles (8.7928, 4.9589) (8.6455, 5.091) (8.6455, 5.2809) knots 0 0 0 1 1 1
  spline S88 degree 2 poles (8.6455, 5.2809) (8.6455, 5.4031) (8.7143, 5.509) knots 0 0 0 1 1 1
  spline S89 degree 2 poles (8.7143, 5.509) (8.7841, 5.616) (8.914, 5.6716) knots 0 0 0 1 1 1
  spline S90 degree 2 poles (8.914, 5.6716) (9.045, 5.7273) (9.2294, 5.7273) knots 0 0 0 1 1 1
  spline S91 degree 2 poles (9.2294, 5.7273) (9.5306, 5.7273) (9.6823, 5.5952) knots 0 0 0 1 1 1
  spline S92 degree 2 poles (9.6823, 5.5952) (9.8351, 5.4632) (9.8428, 5.2427) knots 0 0 0 1 1 1
  line L49 (9.8428, 5.2427) -> (9.5197, 5.2285)
  spline S93 degree 2 poles (9.5197, 5.2285) (9.499, 5.3518) (9.4302, 5.4053) knots 0 0 0 1 1 1
  spline S94 degree 2 poles (9.4302, 5.4053) (9.3626, 5.4599) (9.2261, 5.4599) knots 0 0 0 1 1 1
  spline S95 degree 2 poles (9.2261, 5.4599) (9.0853, 5.4599) (9.0057, 5.402) knots 0 0 0 1 1 1
  spline S96 degree 2 poles (9.0057, 5.402) (8.9544, 5.3649) (8.9544, 5.3027) knots 0 0 0 1 1 1
  spline S97 degree 2 poles (8.9544, 5.3027) (8.9544, 5.246) (9.0024, 5.2056) knots 0 0 0 1 1 1
  spline S98 degree 2 poles (9.0024, 5.2056) (9.0635, 5.1543) (9.2993, 5.0986) knots 0 0 0 1 1 1
  spline S99 degree 2 poles (9.2993, 5.0986) (9.535, 5.043) (9.6474, 4.9829) knots 0 0 0 1 1 1
  spline S100 degree 2 poles (9.6474, 4.9829) (9.7609, 4.924) (9.8242, 4.8203) knots 0 0 0 1 1 1
  spline S101 degree 2 poles (9.8242, 4.8203) (9.8886, 4.7177) (9.8886, 4.566) knots 0 0 0 1 1 1
  spline S102 degree 2 poles (9.8886, 4.566) (9.8886, 4.4285) (9.8122, 4.3085) knots 0 0 0 1 1 1
  spline S103 degree 2 poles (9.8122, 4.3085) (9.7358, 4.1884) (9.5961, 4.1295) knots 0 0 0 1 1 1
  spline S104 degree 2 poles (9.5961, 4.1295) (9.4564, 4.0716) (9.248, 4.0716) knots 0 0 0 1 1 1
  spline S105 degree 2 poles (9.248, 4.0716) (8.9445, 4.0716) (8.7819, 4.2113) knots 0 0 0 1 1 1
  spline S106 degree 2 poles (8.7819, 4.2113) (8.6193, 4.3521) (8.5877, 4.6206) knots 0 0 0 1 1 1
  line L50 (10.9047, 4.6883) -> (10.9047, 4.9578)
  line L51 (10.9047, 4.9578) -> (11.601, 4.9578)
  line L52 (11.601, 4.9578) -> (11.601, 4.3205)
  spline S107 degree 2 poles (11.601, 4.3205) (11.4995, 4.2222) (11.3063, 4.1469) knots 0 0 0 1 1 1
  spline S108 degree 2 poles (11.3063, 4.1469) (11.1143, 4.0727) (10.9167, 4.0727) knots 0 0 0 1 1 1
  spline S109 degree 2 poles (10.9167, 4.0727) (10.6657, 4.0727) (10.4791, 4.1775) knots 0 0 0 1 1 1
  spline S110 degree 2 poles (10.4791, 4.1775) (10.2924, 4.2834) (10.1986, 4.4787) knots 0 0 0 1 1 1
  spline S111 degree 2 poles (10.1986, 4.4787) (10.1047, 4.6752) (10.1047, 4.9055) knots 0 0 0 1 1 1
  spline S112 degree 2 poles (10.1047, 4.9055) (10.1047, 5.1554) (10.2095, 5.3497) knots 0 0 0 1 1 1
  spline S113 degree 2 poles (10.2095, 5.3497) (10.3143, 5.5439) (10.5162, 5.6476) knots 0 0 0 1 1 1
  spline S114 degree 2 poles (10.5162, 5.6476) (10.6701, 5.7273) (10.8993, 5.7273) knots 0 0 0 1 1 1
  spline S115 degree 2 poles (10.8993, 5.7273) (11.1972, 5.7273) (11.3642, 5.6018) knots 0 0 0 1 1 1
  spline S116 degree 2 poles (11.3642, 5.6018) (11.5323, 5.4774) (11.5803, 5.2569) knots 0 0 0 1 1 1
  line L53 (11.5803, 5.2569) -> (11.2594, 5.1969)
  spline S117 degree 2 poles (11.2594, 5.1969) (11.2256, 5.3147) (11.1317, 5.3824) knots 0 0 0 1 1 1
  spline S118 degree 2 poles (11.1317, 5.3824) (11.0389, 5.4512) (10.8993, 5.4512) knots 0 0 0 1 1 1
  spline S119 degree 2 poles (10.8993, 5.4512) (10.6875, 5.4512) (10.562, 5.3169) knots 0 0 0 1 1 1
  spline S120 degree 2 poles (10.562, 5.3169) (10.4376, 5.1827) (10.4376, 4.9186) knots 0 0 0 1 1 1
  spline S121 degree 2 poles (10.4376, 4.9186) (10.4376, 4.6337) (10.5642, 4.4907) knots 0 0 0 1 1 1
  spline S122 degree 2 poles (10.5642, 4.4907) (10.6908, 4.3488) (10.896, 4.3488) knots 0 0 0 1 1 1
  spline S123 degree 2 poles (10.896, 4.3488) (10.9975, 4.3488) (11.099, 4.3881) knots 0 0 0 1 1 1
  spline S124 degree 2 poles (11.099, 4.3881) (11.2016, 4.4285) (11.2747, 4.4853) knots 0 0 0 1 1 1
  line L54 (11.2747, 4.4853) -> (11.2747, 4.6883)
  line L55 (11.2747, 4.6883) -> (10.9047, 4.6883)
  line L56 (11.8379, 4.47) -> (12.1347, 4.5027)
  spline S125 degree 2 poles (12.1347, 4.5027) (12.1456, 4.4121) (12.1915, 4.3685) knots 0 0 0 1 1 1
  spline S126 degree 2 poles (12.1915, 4.3685) (12.2373, 4.3248) (12.3126, 4.3248) knots 0 0 0 1 1 1
  spline S127 degree 2 poles (12.3126, 4.3248) (12.4076, 4.3248) (12.4741, 4.4121) knots 0 0 0 1 1 1
  spline S128 degree 2 poles (12.4741, 4.4121) (12.5407, 4.4995) (12.5593, 4.7745) knots 0 0 0 1 1 1
  spline S129 degree 2 poles (12.5593, 4.7745) (12.4436, 4.6402) (12.2701, 4.6402) knots 0 0 0 1 1 1
  spline S130 degree 2 poles (12.2701, 4.6402) (12.0812, 4.6402) (11.9437, 4.7854) knots 0 0 0 1 1 1
  spline S131 degree 2 poles (11.9437, 4.7854) (11.8073, 4.9317) (11.8073, 5.1652) knots 0 0 0 1 1 1
  spline S132 degree 2 poles (11.8073, 5.1652) (11.8073, 5.4086) (11.9514, 5.557) knots 0 0 0 1 1 1
  spline S133 degree 2 poles (11.9514, 5.557) (12.0965, 5.7065) (12.3203, 5.7065) knots 0 0 0 1 1 1
  spline S134 degree 2 poles (12.3203, 5.7065) (12.5636, 5.7065) (12.7197, 5.5177) knots 0 0 0 1 1 1
  spline S135 degree 2 poles (12.7197, 5.5177) (12.8758, 5.33) (12.8758, 4.8989) knots 0 0 0 1 1 1
  spline S136 degree 2 poles (12.8758, 4.8989) (12.8758, 4.4602) (12.7132, 4.2659) knots 0 0 0 1 1 1
  spline S137 degree 2 poles (12.7132, 4.2659) (12.5505, 4.0716) (12.2897, 4.0716) knots 0 0 0 1 1 1
  spline S138 degree 2 poles (12.2897, 4.0716) (12.102, 4.0716) (11.9863, 4.1709) knots 0 0 0 1 1 1
  spline S139 degree 2 poles (11.9863, 4.1709) (11.8706, 4.2714) (11.8379, 4.47) knots 0 0 0 1 1 1
  spline S140 degree 2 poles (12.532, 5.1401) (12.532, 5.2885) (12.4632, 5.3704) knots 0 0 0 1 1 1
  spline S141 degree 2 poles (12.4632, 5.3704) (12.3956, 5.4523) (12.3061, 5.4523) knots 0 0 0 1 1 1
  spline S142 degree 2 poles (12.3061, 5.4523) (12.2209, 5.4523) (12.1642, 5.3846) knots 0 0 0 1 1 1
  spline S143 degree 2 poles (12.1642, 5.3846) (12.1085, 5.318) (12.1085, 5.1652) knots 0 0 0 1 1 1
  spline S144 degree 2 poles (12.1085, 5.1652) (12.1085, 5.0102) (12.1696, 4.9371) knots 0 0 0 1 1 1
  spline S145 degree 2 poles (12.1696, 4.9371) (12.2308, 4.8651) (12.3224, 4.8651) knots 0 0 0 1 1 1
  spline S146 degree 2 poles (12.3224, 4.8651) (12.4108, 4.8651) (12.4709, 4.9349) knots 0 0 0 1 1 1
  spline S147 degree 2 poles (12.4709, 4.9349) (12.532, 5.0048) (12.532, 5.1401) knots 0 0 0 1 1 1
  spline S148 degree 2 poles (13.5928, 5.7065) (13.8253, 5.7065) (13.9563, 5.5407) knots 0 0 0 1 1 1
  spline S149 degree 2 poles (13.9563, 5.5407) (14.1123, 5.3442) (14.1123, 4.8891) knots 0 0 0 1 1 1
  spline S150 degree 2 poles (14.1123, 4.8891) (14.1123, 4.4351) (13.9552, 4.2364) knots 0 0 0 1 1 1
  spline S151 degree 2 poles (13.9552, 4.2364) (13.8253, 4.0727) (13.5928, 4.0727) knots 0 0 0 1 1 1
  spline S152 degree 2 poles (13.5928, 4.0727) (13.3593, 4.0727) (13.2163, 4.2517) knots 0 0 0 1 1 1
  spline S153 degree 2 poles (13.2163, 4.2517) (13.0733, 4.4318) (13.0733, 4.8924) knots 0 0 0 1 1 1
  spline S154 degree 2 poles (13.0733, 4.8924) (13.0733, 5.3442) (13.2305, 5.5428) knots 0 0 0 1 1 1
  spline S155 degree 2 poles (13.2305, 5.5428) (13.3604, 5.7065) (13.5928, 5.7065) knots 0 0 0 1 1 1
  spline S156 degree 2 poles (13.5928, 5.4523) (13.5372, 5.4523) (13.4935, 5.4162) knots 0 0 0 1 1 1
  spline S157 degree 2 poles (13.4935, 5.4162) (13.4499, 5.3813) (13.4259, 5.2896) knots 0 0 0 1 1 1
  spline S158 degree 2 poles (13.4259, 5.2896) (13.3942, 5.1707) (13.3942, 4.8891) knots 0 0 0 1 1 1
  spline S159 degree 2 poles (13.3942, 4.8891) (13.3942, 4.6075) (13.4226, 4.5016) knots 0 0 0 1 1 1
  spline S160 degree 2 poles (13.4226, 4.5016) (13.451, 4.3969) (13.4935, 4.3619) knots 0 0 0 1 1 1
  spline S161 degree 2 poles (13.4935, 4.3619) (13.5372, 4.327) (13.5928, 4.327) knots 0 0 0 1 1 1
  spline S162 degree 2 poles (13.5928, 4.327) (13.6485, 4.327) (13.6922, 4.3619) knots 0 0 0 1 1 1
  spline S163 degree 2 poles (13.6922, 4.3619) (13.7358, 4.398) (13.7598, 4.4896) knots 0 0 0 1 1 1
  spline S164 degree 2 poles (13.7598, 4.4896) (13.7915, 4.6075) (13.7915, 4.8891) knots 0 0 0 1 1 1
  spline S165 degree 2 poles (13.7915, 4.8891) (13.7915, 5.1707) (13.7631, 5.2754) knots 0 0 0 1 1 1
  spline S166 degree 2 poles (13.7631, 5.2754) (13.7347, 5.3813) (13.6911, 5.4162) knots 0 0 0 1 1 1
  spline S167 degree 2 poles (13.6911, 5.4162) (13.6485, 5.4523) (13.5928, 5.4523) knots 0 0 0 1 1 1
extrude "Extrude14" add sketch "Sketch14" along normal blind 0.05 contours L4 L5 L6 L7 L8 L9 L10 L11 | S0 S1 S2 S3 S4 S5 S6 S7 S8 S9 | L12 L13 L14 L15 L16 L17 L18 L19 L20 L21 L22 L23 L24 | L25 S18 S19 S20 S21 S22 S23 S24 S25 L26 S26 S27 S28 S29 | L28 L29 L30 L31 S34 S35 S36 L32 S37 S38 S39 S40 L33 | L34 L35 S41 S42 S43 S44 S45 S46 S47 L36 L37 L38 | L42 L43 L44 L45 S54 S55 S56 L46 S57 S58 S59 S60 L47 | S61 S62 S63 S64 S65 S66 S67 S68 S69 S70 | L48 S79 S80 S81 S82 S83 S84 S85 S86 S87 S88 S89 S90 S91 S92 L49 S93 S94 S95 S96 S97 S98 S99 S100 S101 S102 S103 S104 S105 S106 | L50 L51 L52 S107 S108 S109 S110 S111 S112 S113 S114 S115 S116 L53 S117 S118 S119 S120 S121 S122 S123 S124 L54 L55 | L56 S125 S126 S127 S128 S129 S130 S131 S132 S133 S134 S135 S136 S137 S138 S139 | S148 S149 S150 S151 S152 S153 S154 S155 bodies 7